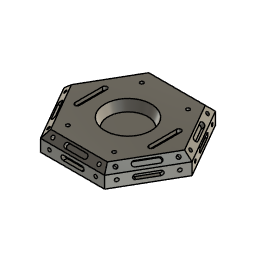
Qatest-Router Test (Autodesk Fusion 360 design; units mm, degrees)
Autodesk Fusion 360 part; units mm, degrees
sketch "Sketch2" plane through (0, 0, 0) normal (0, 0, 1) x (1, 0, 0)
  line L0 (-87.9882, 152.4) -> (-175.9764, 0)
  line L1 (-175.9764, 0) -> (-87.9882, -152.4)
  line L2 (-87.9882, -152.4) -> (87.9882, -152.4)
  line L3 (87.9882, -152.4) -> (175.9764, 0)
  line L4 (175.9764, 0) -> (87.9882, 152.4)
  line L5 (87.9882, 152.4) -> (-87.9882, 152.4)
  dimension "d3" = 152.4
  measures "d3" distance of origin L5
extrude "Extrude1" add sketch "Sketch2" along normal blind 50.8
chamfer "Chamfer1" distance 17.78 angle 45 6 edges at (131.9823, -76.2, 50.8) (0, -152.4, 50.8) (-131.9823, -76.2, 50.8) (-131.9823, 76.2, 50.8) (0, 152.4, 50.8) (131.9823, 76.2, 50.8)
sketch "Sketch3" plane through (0, 0, 50.8) normal (0, 0, 1) x (-1, 0, 0)
  line L0 (77.7229, -134.62) -> (155.4458, 0)
  line L1 (155.4458, 0) -> (77.7229, 134.62)
  line L2 (77.7229, 134.62) -> (-77.7229, 134.62)
  line L3 (-77.7229, 134.62) -> (-155.4458, 0)
  line L4 (-155.4458, 0) -> (-77.7229, -134.62)
  line L5 (-77.7229, -134.62) -> (77.7229, -134.62)
  circle A0 centre (0, 0) radius 63.5
  constraint coincident A0.centre origin
extrude "Extrude2" cut sketch "Sketch3" against normal blind 25.4 draft -20 contours A0
sketch "Sketch4" plane through (0, -152.4, 0) normal (0, -1, 0) x (1, 0, 0)
  line L0 (87.9882, 33.02) -> (-87.9882, 33.02)
  line L1 (-87.9882, 33.02) -> (-87.9882, 0)
  line L2 (-87.9882, 0) -> (87.9882, 0)
  line L3 (87.9882, 0) -> (87.9882, 33.02)
  line L4 (-25.4, 11.43) -> (25.4, 11.43)
  arc A0 (25.4, 11.43) -> (25.4, 24.13) centre (25.4, 17.78) ccw
  line L5 (25.4, 24.13) -> (-25.4, 24.13)
  arc A1 (-25.4, 24.13) -> (-25.4, 11.43) centre (-25.4, 17.78) ccw
  line L6 (-25.4, 17.78) -> (25.4, 17.78) construction
  circle A2 centre (-63.5, 17.78) radius 4.7625
  circle A3 centre (63.5, 17.78) radius 4.7625
  dimension "d11" = 175.9764
  dimension "d12" = 12.7
  dimension "d13" = 9.525
  dimension "d14" = 9.525
  constraint tangent L4 A0
  constraint tangent A0 L5
  constraint parallel L4 L5
  constraint tangent L5 A1
  constraint tangent L4 A1
  constraint horizontal L6
  measures "d11" distance of L1 L3
  measures "d12" diameter of A0
  measures "d13" diameter of A2
  measures "d14" diameter of A3
sketch "Sketch5" plane through (0, -92.71, 92.71) normal (0, -0.707107, 0.707107) x (1, 0, 0)
  line L0 (-87.9882, -84.4144) -> (87.9882, -84.4144)
  line L1 (87.9882, -84.4144) -> (77.7229, -59.2697)
  line L2 (77.7229, -59.2697) -> (-77.7229, -59.2697)
  line L3 (-77.7229, -59.2697) -> (-87.9882, -84.4144)
  line L4 (-25.4, -77.47) -> (25.4, -77.47)
  arc A0 (25.4, -77.47) -> (25.4, -64.77) centre (25.4, -71.12) ccw
  line L5 (25.4, -64.77) -> (-25.4, -64.77)
  arc A1 (-25.4, -64.77) -> (-25.4, -77.47) centre (-25.4, -71.12) ccw
  line L6 (-25.4, -71.12) -> (25.4, -71.12) construction
  circle A2 centre (-63.5, -71.12) radius 4.7625
  circle A3 centre (63.5, -71.12) radius 4.7625
  dimension "d15" = 12.7
  dimension "d16" = 9.525
  dimension "d17" = 9.525
  constraint tangent L4 A0
  constraint tangent A0 L5
  constraint parallel L4 L5
  constraint tangent L5 A1
  constraint tangent L4 A1
  constraint parallel L0 L6
  measures "d15" diameter of A0
  measures "d16" diameter of A2
  measures "d17" diameter of A3
extrude "Extrude3" cut sketch "Sketch5" against normal blind 15.24 contours A2
extrude "Extrude4" cut sketch "Sketch5" against normal blind 15.24 contours A3
extrude "Extrude5" cut sketch "Sketch5" against normal blind 10.16 contours L4 A0 L5 A1
extrude "Extrude6" cut sketch "Sketch4" against normal blind 15.24 contours A2
extrude "Extrude7" cut sketch "Sketch4" against normal blind 10.16 contours L4 A0 L5 A1
extrude "Extrude8" cut sketch "Sketch4" against normal blind 15.24 contours A3
pattern_circular "C-Pattern1" count 6 over 360 about axis through (0, 0, 50.8) along (0, 0, -1) of "Extrude3", "Extrude4", "Extrude5", "Extrude6", "Extrude7", "Extrude8"
sketch "Sketch6" plane through (0, 0, 50.8) normal (0, 0, 1) x (-1, 0, 0)
  circle A0 centre (0, 0) radius 63.5
  line L0 (77.7229, -134.62) -> (155.4458, 0)
  line L1 (155.4458, 0) -> (77.7229, 134.62)
  line L2 (77.7229, 134.62) -> (-77.7229, 134.62)
  line L3 (-77.7229, 134.62) -> (-155.4458, 0)
  line L4 (-155.4458, 0) -> (-77.7229, -134.62)
  line L5 (-77.7229, -134.62) -> (77.7229, -134.62)
  circle A1 centre (63.5, -101.6) radius 4.7625
  circle A2 centre (-63.5, -101.6) radius 4.7625
  circle A3 centre (63.5, 101.6) radius 4.7625
  circle A4 centre (-63.5, 101.6) radius 4.7625
  line L6 (107.95, -38.1) -> (107.95, 38.1)
  arc A5 (107.95, 38.1) -> (95.25, 38.1) centre (101.6, 38.1) ccw
  line L7 (95.25, 38.1) -> (95.25, -38.1)
  arc A6 (95.25, -38.1) -> (107.95, -38.1) centre (101.6, -38.1) ccw
  line L8 (101.6, -38.1) -> (101.6, 38.1) construction
  line L9 (-95.25, -38.1) -> (-95.25, 38.1)
  arc A7 (-95.25, 38.1) -> (-107.95, 38.1) centre (-101.6, 38.1) ccw
  line L10 (-107.95, 38.1) -> (-107.95, -38.1)
  arc A8 (-107.95, -38.1) -> (-95.25, -38.1) centre (-101.6, -38.1) ccw
  line L11 (-101.6, -38.1) -> (-101.6, 38.1) construction
  dimension "d32" = 9.525
  dimension "d33" = 9.525
  dimension "d34" = 9.525
  dimension "d35" = 9.525
  dimension "d38" = 12.7
  dimension "d39" = 12.7
  constraint tangent L6 A5
  constraint tangent A5 L7
  constraint parallel L6 L7
  constraint tangent L7 A6
  constraint tangent L6 A6
  constraint vertical L8
  constraint tangent L9 A7
  constraint tangent A7 L10
  constraint parallel L9 L10
  constraint tangent L10 A8
  constraint tangent L9 A8
  constraint perpendicular L5 L11
  measures "d32" diameter of A1
  measures "d33" diameter of A2
  measures "d34" diameter of A3
  measures "d35" diameter of A4
  measures "d38" diameter of A5
  measures "d39" diameter of A7
extrude "Extrude9" cut sketch "Sketch6" against normal blind 25.4 contours A1 | A2 | A3 | A4
extrude "Extrude10" cut sketch "Sketch6" against normal blind 10.16 contours L6 A5 L7 A6 | L9 A7 L10 A8
equation "Cone_Taper = 20 in"
